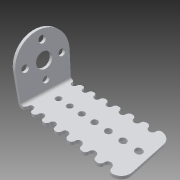
# Autodesk Inventor part: Brida Sujección Motor
Saved by Autodesk Inventor 2014 (Build 180170000, 170)
## iProperties
Created: 2014-01-26
Part Number: Brida Sujección Motor
Material: Aluminio-6061
Document SubType Name: Modeling
Designer: Sanjo
Mass: 6.9891 g
Surface Area: 38.8646 cm^2
Volume: 2.579 cm^3
Density: 2.71 g/cm^3
Appearance: Aluminio - Oscuro
Author: Sanjo
Autodesk Inventor part; units mm, degrees
ref_plane "YZ Plane" through (0, 0, 0) normal (1, 0, 0) x (0, 1, 0)
ref_plane "XZ Plane" through (0, 0, 0) normal (0, 1, 0) x (-1, 0, 0)
ref_plane "XY Plane" through (0, 0, 0) normal (0, 0, 1) x (1, 0, 0)
sketch "Boceto2" plane through (0, 0, 0) normal (1, 0, 0) x (0, 1, 0)
  circle A0 centre (0, 0) radius 3.75
  arc A1 (12.5, 0) -> (-12.5, 0) centre (0, 0) ccw
  line L0 (-12.5, 0) -> (-12.5, -14)
  line L1 (12.5, 0) -> (12.5, -14)
  line L2 (-12.5, -14) -> (12.5, -14)
  circle A2 centre (0, 8.5) radius 1.65
  circle A3 centre (-8.5, 0) radius 1.65
  circle A4 centre (0, -8.5) radius 1.65
  circle A5 centre (8.5, 0) radius 1.65
  dimension "d2" = 7.5
  dimension "d3" = 25
  dimension "d4" = 14
  dimension "d5" = 14
  dimension "d10" = 3.3
  dimension "d13" = 360
  constraints: 6 centre point, 6 end point, 2 coincident, 2 point on circle, 2 tangent, 1 parallel, 1 vertical, 9 other
  measures "d2" diameter of A0
  measures "d3" diameter of A1
  measures "d4" distance of L0.start L0.end
  measures "d5" distance of L1.start L1.end
  measures "d10" diameter of A2
extrude "Extrusión2" add sketch "Boceto2" against normal blind 1.5
sketch "Boceto4" plane through (0, -12.5, -14) normal (0, 0, -1) x (-1, 0, 0)
  line L0 (-49, 0) -> (-49, 25)
  line L1 (-49, 25) -> (-45.2, 25)
  line L2 (1.5, 0) -> (1.5, 25) projected
  line L3 (0, 25) -> (1.5, 25) projected
  line L4 (0, 0) -> (1.5, 0) projected
  circle A0 centre (-6.8, 12.5) radius 1.5
  circle A1 centre (-13.2, 12.5) radius 1.5
  circle A2 centre (-19.6, 12.5) radius 1.5
  circle A3 centre (-26, 12.5) radius 1.5
  circle A4 centre (-32.4, 12.5) radius 1.5
  circle A5 centre (-38.8, 12.5) radius 1.5
  circle A6 centre (-45.2, 12.5) radius 1.5
  arc A7 (-40.7, 1.5) -> (-43.7, 1.5) centre (-42.2, 1.5) ccw
  arc A8 (-43.7, 23.5) -> (-40.7, 23.5) centre (-42.2, 23.5) ccw
  line L5 (-43.7, 23.5) -> (-43.7, 23.5)
  line L6 (-40.7, 23.5) -> (-40.7, 23.5)
  arc A9 (-37.3, 23.5) -> (-34.3, 23.5) centre (-35.8, 23.5) ccw
  line L7 (-37.3, 23.5) -> (-37.3, 23.5)
  line L8 (-34.3, 23.5) -> (-34.3, 23.5)
  arc A10 (-30.9, 23.5) -> (-27.9, 23.5) centre (-29.4, 23.5) ccw
  line L9 (-30.9, 23.5) -> (-30.9, 23.5)
  line L10 (-27.9, 23.5) -> (-27.9, 23.5)
  arc A11 (-24.5, 23.5) -> (-21.5, 23.5) centre (-23, 23.5) ccw
  line L11 (-24.5, 23.5) -> (-24.5, 23.5)
  line L12 (-21.5, 23.5) -> (-21.5, 23.5)
  arc A12 (-18.1, 23.5) -> (-15.1, 23.5) centre (-16.6, 23.5) ccw
  line L13 (-18.1, 23.5) -> (-18.1, 23.5)
  line L14 (-15.1, 23.5) -> (-15.1, 23.5)
  arc A13 (-11.7, 23.5) -> (-8.7, 23.5) centre (-10.2, 23.5) ccw
  line L15 (-11.7, 23.5) -> (-11.7, 23.5)
  line L16 (-8.7, 23.5) -> (-8.7, 23.5)
  arc A14 (-5.3, 23.5) -> (-2.3, 23.5) centre (-3.8, 23.5) ccw
  line L17 (-5.3, 23.5) -> (-5.3, 23.5)
  line L18 (-2.3, 23.5) -> (-2.3, 23.5)
  line L19 (-43.7, 1.5) -> (-43.7, 1.5)
  line L20 (-40.7, 1.5) -> (-40.7, 1.5)
  arc A15 (-34.3, 1.5) -> (-37.3, 1.5) centre (-35.8, 1.5) ccw
  line L21 (-37.3, 1.5) -> (-37.3, 1.5)
  line L22 (-34.3, 1.5) -> (-34.3, 1.5)
  arc A16 (-27.9, 1.5) -> (-30.9, 1.5) centre (-29.4, 1.5) ccw
  line L23 (-30.9, 1.5) -> (-30.9, 1.5)
  line L24 (-27.9, 1.5) -> (-27.9, 1.5)
  arc A17 (-21.5, 1.5) -> (-24.5, 1.5) centre (-23, 1.5) ccw
  line L25 (-24.5, 1.5) -> (-24.5, 1.5)
  line L26 (-21.5, 1.5) -> (-21.5, 1.5)
  arc A18 (-15.1, 1.5) -> (-18.1, 1.5) centre (-16.6, 1.5) ccw
  line L27 (-18.1, 1.5) -> (-18.1, 1.5)
  line L28 (-15.1, 1.5) -> (-15.1, 1.5)
  arc A19 (-8.7, 1.5) -> (-11.7, 1.5) centre (-10.2, 1.5) ccw
  line L29 (-11.7, 1.5) -> (-11.7, 1.5)
  line L30 (-8.7, 1.5) -> (-8.7, 1.5)
  arc A20 (-2.3, 1.5) -> (-5.3, 1.5) centre (-3.8, 1.5) ccw
  line L31 (-5.3, 1.5) -> (-5.3, 1.5)
  line L32 (-2.3, 1.5) -> (-2.3, 1.5)
  line L33 (-45.2, 0) -> (-49, 0)
  line L34 (-38.8, 0) -> (-39.2, 0)
  line L35 (-32.4, 0) -> (-32.8, 0)
  line L36 (-26, 0) -> (-26.4, 0)
  line L37 (-19.6, 0) -> (-20, 0)
  line L38 (-13.2, 0) -> (-13.6, 0)
  line L39 (0, 0) -> (-0.8, 0)
  line L40 (-6.8, 0) -> (-7.2, 0)
  arc A21 (-45.2, 0) -> (-43.7, 1.5) centre (-45.2, 1.5) ccw
  arc A22 (-40.7, 1.5) -> (-39.2, 0) centre (-39.2, 1.5) ccw
  arc A23 (-38.8, 0) -> (-37.3, 1.5) centre (-38.8, 1.5) ccw
  arc A24 (-34.3, 1.5) -> (-32.8, 0) centre (-32.8, 1.5) ccw
  arc A25 (-32.4, 0) -> (-30.9, 1.5) centre (-32.4, 1.5) ccw
  arc A26 (-27.9, 1.5) -> (-26.4, 0) centre (-26.4, 1.5) ccw
  arc A27 (-26, 0) -> (-24.5, 1.5) centre (-26, 1.5) ccw
  arc A28 (-21.5, 1.5) -> (-20, 0) centre (-20, 1.5) ccw
  arc A29 (-19.6, 0) -> (-18.1, 1.5) centre (-19.6, 1.5) ccw
  arc A30 (-15.1, 1.5) -> (-13.6, 0) centre (-13.6, 1.5) ccw
  arc A31 (-13.2, 0) -> (-11.7, 1.5) centre (-13.2, 1.5) ccw
  arc A32 (-8.7, 1.5) -> (-7.2, 0) centre (-7.2, 1.5) ccw
  arc A33 (-6.8, 0) -> (-5.3, 1.5) centre (-6.8, 1.5) ccw
  arc A34 (-2.3, 1.5) -> (-0.8, 0) centre (-0.8, 1.5) ccw
  arc A35 (-43.7, 23.5) -> (-45.2, 25) centre (-45.2, 23.5) ccw
  line L41 (-39.2, 25) -> (-38.8, 25)
  line L42 (-32.8, 25) -> (-32.4, 25)
  line L43 (-26.4, 25) -> (-26, 25)
  line L44 (-20, 25) -> (-19.6, 25)
  line L45 (-13.6, 25) -> (-13.2, 25)
  line L46 (-7.2, 25) -> (-6.8, 25)
  line L47 (-0.8, 25) -> (0, 25)
  arc A36 (-5.3, 23.5) -> (-6.8, 25) centre (-6.8, 23.5) ccw
  arc A37 (-7.2, 25) -> (-8.7, 23.5) centre (-7.2, 23.5) ccw
  arc A38 (-13.6, 25) -> (-15.1, 23.5) centre (-13.6, 23.5) ccw
  arc A39 (-18.1, 23.5) -> (-19.6, 25) centre (-19.6, 23.5) ccw
  arc A40 (-20, 25) -> (-21.5, 23.5) centre (-20, 23.5) ccw
  arc A41 (-24.5, 23.5) -> (-26, 25) centre (-26, 23.5) ccw
  arc A42 (-26.4, 25) -> (-27.9, 23.5) centre (-26.4, 23.5) ccw
  arc A43 (-30.9, 23.5) -> (-32.4, 25) centre (-32.4, 23.5) ccw
  arc A44 (-32.8, 25) -> (-34.3, 23.5) centre (-32.8, 23.5) ccw
  arc A45 (-37.3, 23.5) -> (-38.8, 25) centre (-38.8, 23.5) ccw
  arc A46 (-39.2, 25) -> (-40.7, 23.5) centre (-39.2, 23.5) ccw
  arc A47 (-11.7, 23.5) -> (-13.2, 25) centre (-13.2, 23.5) ccw
  arc A48 (-0.8, 25) -> (-2.3, 23.5) centre (-0.8, 23.5) ccw
  line L48 (0, 0) -> (1.5, 0)
  line L49 (1.5, 25) -> (0, 25)
  point P0 (0, 12.5)
  point P1 (-43.7, 25)
  point P2 (-40.7, 25)
  point P3 (-43.7, 0)
  point P4 (-40.7, 0)
  point P5 (-37.3, 0)
  point P6 (-34.3, 0)
  point P7 (-30.9, 0)
  point P8 (-27.9, 0)
  point P9 (-24.5, 0)
  point P10 (-21.5, 0)
  point P11 (-18.1, 0)
  point P12 (-15.1, 0)
  point P13 (-11.7, 0)
  point P14 (-8.7, 0)
  point P15 (-5.3, 0)
  point P16 (-2.3, 0)
  dimension "d29" = 49
  dimension "d32" = 3
  dimension "d33" = 8.3
  dimension "d36" = 6.4
  dimension "d63" = 3
  dimension "d74" = 3
  dimension "d79" = 3
  dimension "d84" = 3
  dimension "d89" = 3
  dimension "d94" = 3
  dimension "d99" = 3
  dimension "d104" = 3
  dimension "d109" = 3
  dimension "d114" = 3
  dimension "d119" = 3
  dimension "d124" = 3
  dimension "d129" = 3
  dimension "d134" = 3
  dimension "d135" = 1.5
  dimension "d136" = 1.5
  dimension "d137" = 1.5
  dimension "d138" = 1.5
  dimension "d139" = 1.5
  dimension "d140" = 1.5
  dimension "d141" = 1.5
  dimension "d142" = 1.5
  dimension "d143" = 1.5
  dimension "d144" = 1.5
  dimension "d145" = 1.5
  dimension "d146" = 1.5
  dimension "d147" = 1.5
  dimension "d148" = 1.5
  dimension "d149" = 1.5
  dimension "d150" = 1.5
  dimension "d151" = 1.5
  constraints: 94 end point, 84 point on circle, 84 tangent, 49 centre point, 34 point on line, 11 equal radius, 10 parallel, 10 perpendicular, 7 collinear, 1 horizontal, 12 other
  measures "d29" distance from line of point (0, 12.5) L0
  measures "d32" diameter of A0
  measures "d33" distance from line of L2 A0.centre
  measures "d36" distance of A0.centre A1.centre
  measures "d63" diameter of A7
  measures "d74" diameter of A8
  measures "d79" diameter of A9
  measures "d84" diameter of A10
  measures "d89" diameter of A11
  measures "d94" diameter of A12
  measures "d99" diameter of A13
  measures "d104" diameter of A14
  measures "d109" diameter of A15
  measures "d114" diameter of A16
  measures "d119" diameter of A17
  measures "d124" diameter of A18
  measures "d129" diameter of A19
  measures "d134" diameter of A20
  measures "d135" radius of A21
  measures "d136" radius of A22
  measures "d137" radius of A23
  measures "d138" radius of A24
  measures "d139" radius of A25
  measures "d140" radius of A26
  measures "d141" radius of A27
  measures "d142" radius of A28
  measures "d143" radius of A29
  measures "d144" radius of A30
  measures "d145" radius of A31
  measures "d146" radius of A32
  measures "d147" radius of A33
  measures "d148" radius of A34
  measures "d149" radius of A35
  measures "d150" radius of A36
  measures "d151" radius of A47
extrude "Extrusión4" add sketch "Boceto4" along normal blind 1.5
fillet "Empalme1" radius 1.5 2 edges at (0, 0, -14) (-1.5, 0, -15.5)
fillet "Empalme2" radius 4.6 2 edges at (49, -12.5, -14.75) (49, 12.5, -14.75)
